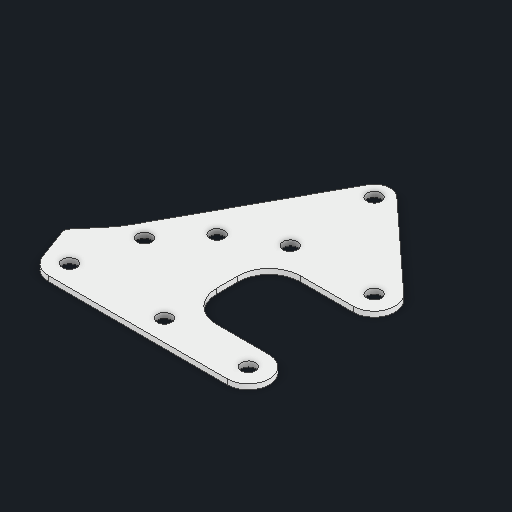
# Autodesk Inventor part: Funnel Gusset Back Improved
Saved by Autodesk Inventor 2025.1 (Build 291241000, 241)
## iProperties
Created: 2024-10-23
Part Number: Funnel Gusset Back Improved
Material: Acetal Resin, White
Document SubType Name: Modeling
Designer: avere
Density: 1.425 g/cm^3
Appearance: Smooth - White
Author: avere
Autodesk Inventor part; units mm, degrees
ref_plane "YZ Plane" through (0, 0, 0) normal (1, 0, 0) x (0, 1, 0)
ref_plane "XZ Plane" through (0, 0, 0) normal (0, 1, 0) x (-1, 0, 0)
ref_plane "XY Plane" through (0, 0, 0) normal (0, 0, 1) x (1, 0, 0)
sketch "main" plane through (0, 0, 0) normal (0, 0, 1) x (1, 0, 0)
  line L0 (12.0188, -14.2552) -> (37.3756, 32.0398)
  circle A0 centre (21.7688, 21.6141) radius 2.1844
  line L1 (40.1954, 36.1649) -> (45.6883, 42.7111)
  circle A1 centre (31.8098, 33.5805) radius 2.1844
  circle A2 centre (36.488, 51.5844) radius 2.1844
  arc A3 (42.4433, 53.7882) -> (36.4888, 57.9344) centre (36.488, 51.5844) ccw
  line L2 (45.961, 44.2825) -> (42.4433, 53.7882)
  arc A4 (45.6883, 42.7111) -> (45.961, 44.2825) centre (44.4722, 43.7316) ccw
  line L3 (36.4888, 57.9344) -> (-17.6519, 57.9412)
  circle A5 centre (7.7473, 51.5844) radius 2.1844
  line L4 (7.7515, 35.7094) -> (7.7532, 29.3619)
  arc A6 (7.7515, 35.7094) -> (-1.776, 45.2318) centre (-1.7735, 35.7068) ccw
  arc A7 (-1.7718, 19.8344) -> (7.7532, 29.3619) centre (-1.7718, 29.3594) ccw
  line L5 (-17.651, 45.2276) -> (-1.776, 45.2318)
  arc A8 (-17.6519, 57.9412) -> (-17.651, 45.2276) centre (-17.6527, 51.5844) ccw
  arc A9 (-17.6527, 19.8344) -> (-21.9541, 8.8131) centre (-17.6527, 13.4844) ccw
  circle A10 centre (7.7473, 13.4844) radius 2.1844
  line L6 (-1.7718, 19.8344) -> (-17.6527, 19.8344)
  arc A11 (4.4483, -15.4983) -> (12.0188, -14.2552) centre (7.7473, -11.9156) ccw
  line L7 (4.4483, -15.4983) -> (-21.9541, 8.8131)
  circle A12 centre (7.7473, -11.9156) radius 2.1844
  circle A13 centre (-17.6527, 51.5844) radius 2.1844
  circle A14 centre (-17.6527, 13.4844) radius 2.1844
  arc A15 (40.1954, 36.1649) -> (37.3756, 32.0398) centre (59.6529, 19.8381) ccw
  point P0 (10.5119, 26.5593)
  dimension "d1" = 9.7405
  dimension "d2" = 4.3688
  dimension "d3" = 4.3688
  dimension "d4" = 4.3688
  dimension "d5" = 4.3688
  dimension "d6" = 4.3688
  dimension "d7" = 25.4
  measures "d1" diameter of A11
  measures "d2" diameter of A2
  measures "d3" diameter of A5
  measures "d4" diameter of A1
  measures "d5" diameter of A0
  measures "d6" diameter of A10
  measures "d7" radius of A15
sketch "Sketch1" plane through (0, 0, 0) normal (0, 1, 0) x (-1, 0, 0)
  line L0 (29.6715, -65.8396) -> (55.0283, -19.5445)
  circle A0 centre (39.4215, -29.9702) radius 2.1844
  line L1 (57.8481, -15.4195) -> (63.341, -8.8732)
  circle A1 centre (49.4625, -18.0039) radius 2.1844
  circle A2 centre (54.1407, 0) radius 2.1844
  arc A3 (60.096, 2.2039) -> (54.1415, 6.35) centre (54.1407, 0) ccw
  line L2 (63.6138, -7.3019) -> (60.096, 2.2039)
  arc A4 (63.341, -8.8732) -> (63.6138, -7.3019) centre (62.1249, -7.8528) ccw
  line L3 (54.1415, 6.35) -> (0.0008, 6.3568)
  circle A5 centre (25.4, 0) radius 2.1844
  line L4 (25.4043, -15.875) -> (25.406, -22.2224)
  arc A6 (25.4043, -15.875) -> (15.8767, -6.3526) centre (15.8793, -15.8776) ccw
  arc A7 (15.881, -31.75) -> (25.406, -22.2224) centre (15.881, -22.225) ccw
  line L5 (0.0017, -6.3568) -> (15.8767, -6.3526)
  arc A8 (0.0008, 6.3568) -> (0.0017, -6.3568) centre (0, 0) ccw
  arc A9 (0, -31.75) -> (-4.3013, -42.7713) centre (0, -38.1) ccw
  circle A10 centre (25.4, -38.1) radius 2.1844
  line L6 (15.881, -31.75) -> (0, -31.75)
  arc A11 (22.101, -67.0827) -> (29.6715, -65.8396) centre (25.4, -63.5) ccw
  line L7 (22.101, -67.0827) -> (-4.3013, -42.7713)
  circle A12 centre (25.4, -63.5) radius 2.1844
  circle A13 centre (0, 0) radius 2.1844
  circle A14 centre (0, -38.1) radius 2.1844
  arc A15 (57.8481, -15.4195) -> (55.0283, -19.5445) centre (77.3056, -31.7463) ccw
  constraints: 2 other
extrude "Extrusion1" add sketch "Sketch1" along normal blind 1.5875
body "Solid1"
